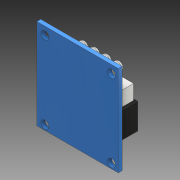
# Autodesk Inventor part: STEPPER DRIVER
Saved by Autodesk Inventor 2017 (Build 210142000, 142)
## iProperties
Created: 2017-04-01
Part Number: STEPPER DRIVER
Material: Generic
Document SubType Name: Modeling
Designer: Muchen
Density: 1 g/cm^3
Appearance: Default
Author: Muchen
Autodesk Inventor part; units mm, degrees
ref_plane "YZ Plane" through (0, 0, 0) normal (1, 0, 0) x (0, 1, 0)
ref_plane "XZ Plane" through (0, 0, 0) normal (0, 1, 0) x (-1, 0, 0)
ref_plane "XY Plane" through (0, 0, 0) normal (0, 0, 1) x (1, 0, 0)
sketch "Sketch1" plane through (0, 0, 0) normal (0, 1, 0) x (-1, 0, 0)
  line L0 (0, 0) -> (-31.55, 0)
  line L1 (-31.55, 0) -> (-31.55, -35)
  line L2 (-31.55, -35) -> (0, -35)
  line L3 (0, -35) -> (0, 0)
  circle A0 centre (-3.15, -33) radius 1.5
  circle A1 centre (-28.95, -33) radius 1.5
  circle A2 centre (-3.15, -3) radius 1.5
  circle A3 centre (-28.95, -3) radius 1.5
  dimension "d0" = 31.55
  dimension "d1" = 35
  dimension "d2" = 3
  dimension "d3" = 25.8
  dimension "d4" = 2.6
  dimension "d5" = 30
  dimension "d6" = 2
  constraints: 8 end point, 4 centre point, 3 equal radius, 2 horizontal alignment, 2 parallel, 2 vertical alignment, 1 horizontal, 1 perpendicular
  measures "d0" distance of L0.start L0.end
  measures "d1" distance of L0.end L1.end
  measures "d2" diameter of A3
  measures "d3" distance of A1.centre A0.centre
  measures "d4" distance from line of L1 A1.centre
  measures "d5" distance of A3.centre A1.centre
  measures "d6" distance from line of L2 A1.centre
extrude "Extrusion1" add sketch "Sketch1" along normal blind 1.5
sketch "Sketch2" plane through (0, 1.5, 0) normal (0, 1, 0) x (1, 0, 0)
  line L0 (9.15, 26.76) -> (29.55, 26.76)
  line L1 (29.55, 26.76) -> (29.55, 16.76)
  line L2 (29.55, 16.76) -> (9.15, 16.76)
  line L3 (9.15, 16.76) -> (9.15, 26.76)
  line L4 (31.55, 35) -> (0, 35) projected
  line L5 (29.05, 16.16) -> (14.05, 16.16)
  line L6 (14.05, 16.16) -> (14.05, 10.45)
  line L7 (14.05, 10.45) -> (29.05, 10.45)
  line L8 (29.05, 10.45) -> (29.05, 16.16)
  line L9 (28.3, 11.2) -> (14.8, 11.2)
  line L10 (14.8, 11.2) -> (14.8, 15.41)
  line L11 (14.8, 15.41) -> (28.3, 15.41)
  line L12 (28.3, 15.41) -> (28.3, 11.2)
  line L13 (31.55, 0) -> (31.55, 35) projected
  circle A0 centre (11.55, 5.6) radius 1.75
  circle A1 centre (16.05, 5.6) radius 1.75
  circle A2 centre (20.55, 5.6) radius 1.75
  circle A3 centre (25.05, 5.6) radius 1.75
  line L14 (0, 0) -> (31.55, 0) projected
  dimension "d9" = 10
  dimension "d10" = 20.4
  dimension "d11" = 8.24
  dimension "d12" = 2
  dimension "d15" = 15
  dimension "d16" = 5.71
  dimension "d17" = 2.5
  dimension "d18" = 10.45
  dimension "d19" = 0.75
  dimension "d22" = 4.5
  dimension "d23" = 4.5
  dimension "d24" = 4.5
  dimension "d25" = 6.5
  dimension "d26" = 5.6
  dimension "d27" = 3.5
  constraints: 24 end point, 6 parallel, 4 centre point, 3 equal radius, 3 horizontal alignment, 3 perpendicular, 2 horizontal, 3 other
  measures "d9" distance of L0.end L1.end
  measures "d10" distance of L1.end L2.end
  measures "d11" distance between parallel lines of L4 L0
  measures "d12" distance from line of L4.start L1
  measures "d15" distance of L6.end L7.end
  measures "d16" distance of L7.end L5.start
  measures "d17" distance between parallel lines of L13 L8
  measures "d18" distance from line of L13.start L7
  measures "d19" distance between parallel lines of L7 L9
  measures "d22" distance of A2.centre A3.centre
  measures "d23" distance of A1.centre A2.centre
  measures "d24" distance of A1.centre A0.centre
  measures "d25" distance from line of L13 A3.centre
  measures "d26" distance from line of L14 A3.centre
  measures "d27" diameter of A2
extrude "Extrusion2" add sketch "Sketch2" along normal blind 8.11 contours L0 L1 L2 L3
extrude "Extrusion3" add sketch "Sketch2" along normal blind 6.9 contours L8 L7 L6 L5
extrude "Extrusion4" add sketch "Sketch2" along normal blind 5.6 contours A0 | A1 | A2 | A3
fillet "Fillet1" radius 1 4 edges at (9.8, 7.1, -5.6) (14.3, 7.1, -5.6) (18.8, 7.1, -5.6) (23.3, 7.1, -5.6)
body "Solid1"
